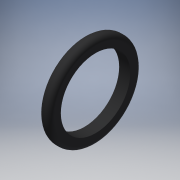
# Autodesk Inventor part: BackWheel
Saved by Autodesk Inventor 2018 (Build 220112000, 112)
## iProperties
Created: 2017-11-19
Part Number: BackWheel
Material: Generic
Document SubType Name: Modeling
Designer: eroldan
Density: 1 g/cm^3
Appearance: Rubber - Black
Author: eroldan
Autodesk Inventor part; units mm, degrees
ref_plane "YZ Plane" through (0, 0, 0) normal (1, 0, 0) x (0, 1, 0)
ref_plane "XZ Plane" through (0, 0, 0) normal (0, 1, 0) x (-1, 0, 0)
ref_plane "XY Plane" through (0, 0, 0) normal (0, 0, 1) x (1, 0, 0)
sketch "Sketch3" plane through (0, 0, 0) normal (0, 0, 1) x (1, 0, 0)
  line L0 (-37.5, 235) -> (37.5, 235)
  line L1 (37.5, 235) -> (37.5, 310)
  line L2 (37.5, 310) -> (-37.5, 310)
  line L3 (-37.5, 310) -> (-37.5, 235)
  line L4 (-37.5, 235) -> (37.5, 310) construction
  line L5 (37.5, 235) -> (-37.5, 310) construction
  line L6 (-52.5, 0) -> (52.5, 0) projected
  point P0 (0, 0)
  point P1 (0, 272.5)
  dimension "d48" = 75
  dimension "d49" = 75
  dimension "d50" = 310
  constraints: 12 end point, 2 midpoint, 2 parallel, 1 horizontal, 1 perpendicular
  measures "d48" distance of L2.end L1.end
  measures "d49" distance of L1.end L0.end
  measures "d50" distance from line of point (0, 0) L2
revolve "Revolution2" add sketch "Sketch3" angle 360 about axis through (-10, 0, 0) along (1, 0, 0)
fillet "Fillet1" radius 30 2 edges at (37.5, -310, 0) (-37.5, -310, 0)
body "Solid1"
